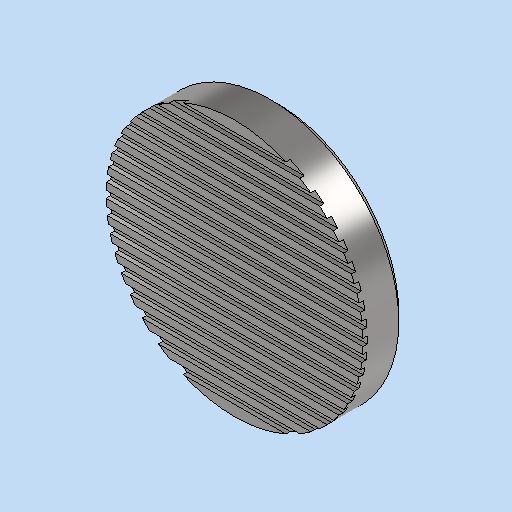
# Autodesk Inventor part: boron-target-grooved
Saved by Autodesk Inventor 2025 (Build 290162000, 162)
## iProperties
Created: 2024-12-16
Part Number: boron-target-grooved
Material: Stainless Steel
Document SubType Name: Modeling
Designer: kuzmin
Density: 8 g/cm^3
Appearance: Semi-Polished
Author: kuzmin
Autodesk Inventor part; units mm, degrees
ref_plane "YZ Plane" through (0, 0, 0) normal (1, 0, 0) x (0, 1, 0)
ref_plane "XZ Plane" through (0, 0, 0) normal (0, 1, 0) x (-1, 0, 0)
ref_plane "XY Plane" through (0, 0, 0) normal (0, 0, 1) x (1, 0, 0)
sketch "Sketch1" plane through (0, 0, 0) normal (0, 0, 1) x (1, 0, 0)
  circle A0 centre (0, 0) radius 9
  dimension "d0" = 18
  constraints: 1 centre point, 1 coincident
  measures "d0" diameter of A0
extrude "Extrusion1" add sketch "Sketch1" along normal blind 3
sketch "Sketch2" plane through (0, 0, 0) normal (1, 0, 0) x (0, 1, 0)
  line L0 (-0.25, 4) -> (0.25, 4)
  line L1 (0.25, 4) -> (0.25, 2.7)
  line L2 (0.25, 2.7) -> (-0.25, 2.7)
  line L3 (-0.25, 2.7) -> (-0.25, 4)
  line L4 (9, 3) -> (-9, 3) projected
  point P0 (0, 0)
  point P1 (0, 4)
  dimension "d3" = 0.5
  dimension "d4" = 1
  dimension "d5" = 0.3
  constraints: 8 end point, 2 parallel, 1 horizontal, 1 midpoint, 1 perpendicular, 1 vertical alignment
  measures "d3" distance of L0.start L0.end
  measures "d4" distance between parallel lines of L4 L0
  measures "d5" distance between parallel lines of L4 L2
extrude "Extrusion2" cut sketch "Sketch2" along normal through all both and the other way through all
pattern_linear "Rectangular Pattern1" count 17 spacing 1 along (0, 1, 0) of "Extrusion2" first direction both ways yes
chamfer "Chamfer1" distance 0.5 angle 45 1 edges at (-9, 0, 0)
body "Solid1"
